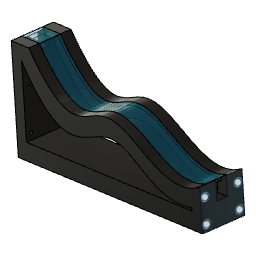
Light Fight Enclosurev2 (Autodesk Fusion 360 archive; units mm, degrees)
design "curvy ramp v4"
Autodesk Fusion 360 part; units mm, degrees
sketch "Sketch1" plane through (0, 0, 0) normal (0, 0, 1) x (1, 0, 0)
  spline S0 degree 5 poles (40.5611, 35.8703) (42.6613, 34.7671) (46.8791, 32.8536) (53.2584, 30.8623) (61.8698, 29.9771) (72.8022, 31.7845) (83.8683, 36.2451) (94.9958, 42.7502) (106.047, 50.0933) (116.8416, 56.5913) (127.2385, 60.6523) (137.2101, 61.2633) (146.9114, 58.4588) (156.7874, 54.0175) (167.5021, 51.0733) (179.7981, 53.3109) (191.4637, 62.1139) (201.4823, 73.9015) (208.7561, 84.2233) (212.5417, 90) knots 0 0 0 0 0 0 0.066667 0.133333 0.2 0.266667 0.333333 0.4 0.466667 0.533333 0.6 0.666667 0.733333 0.8 0.866667 0.933333 1 1 1 1 1 1
  line L0 (179.6056, 39.7401) -> (245.4778, 140.2599)
  line L1 (220.9765, 77.3947) -> (220.9765, 14.5028)
  line L2 (220.9765, 14.5028) -> (50.4348, 14.5028)
  line L3 (40.5611, -0.1297) -> (230.5611, -0.1297)
  line L4 (230.5611, -0.1297) -> (230.5611, 90)
  line L5 (230.5611, 90) -> (220.5417, 90)
  line L6 (212.5417, 90) -> (220.5417, 90)
  line L7 (40.5611, -0.1297) -> (40.5611, 35.8703)
  line L8 (50.4348, 25) -> (50.4348, 29.3921)
  line L9 (45.8578, 33.4692) -> (45.8578, 30.6235)
  spline S1 degree 5 poles (50.4348, 19.7514) (52.5108, 19.1803) (56.647, 18.3263) (62.8042, 17.9102) (70.9306, 19.0395) (81.008, 22.9144) (91.0643, 28.6518) (101.1393, 35.3853) (111.2165, 41.8888) (121.2381, 46.7548) (131.17, 48.8392) (141.0534, 47.6422) (151.0639, 43.7411) (161.5707, 39.2349) (173.0583, 37.1534) (186.051, 40.8954) (198.0379, 51.1114) (208.0885, 63.9297) (215.2808, 74.9049) (219, 81) knots 0 0 0 0 0 0 0.066667 0.133333 0.2 0.266667 0.333333 0.4 0.466667 0.533333 0.6 0.666667 0.733333 0.8 0.866667 0.933333 1 1 1 1 1 1
  line L10 (32.1895, 24.771) -> (68.6802, 14.7318)
  line L11 (195.2279, 42.0418) -> (242.7721, 119.9582)
  spline S2 degree 5 poles (50.4348, 16.9226) (52.4566, 16.5812) (56.4561, 16.0582) (62.3233, 15.7536) (69.8813, 16.311) (78.8871, 18.5852) (87.4629, 22.3093) (95.6403, 27.1967) (103.4817, 32.7308) (111.0884, 38.1119) (118.5816, 42.4668) (126.0845, 45.0565) (133.7053, 45.4599) (141.516, 43.8367) (149.5484, 40.9252) (157.8085, 37.7615) (166.2855, 35.4806) (174.9622, 35.0844) (183.8241, 37.2318) (192.8599, 42.3179) (202.0608, 50.5417) (209.5491, 59.6846) (215.2356, 67.9819) (219.0577, 74.1509) (220.9765, 77.3947) knots 0 0 0 0 0 0 0.05 0.1 0.15 0.2 0.25 0.3 0.35 0.4 0.45 0.5 0.55 0.6 0.65 0.7 0.75 0.8 0.85 0.9 0.95 1 1 1 1 1 1
  line L12 (50.4348, 14.5028) -> (50.4348, 16.9226)
  line L13 (50.4348, 19.7514) -> (50.4348, 25)
  line L14 (215.1059, 87.8623) -> (225.0015, 87.8623)
  line L15 (219, 87.8623) -> (219, 81)
  spline S3 degree 5 poles (45.8578, 30.6235) (46.8345, 30.3152) (48.8626, 29.7261) (51.9972, 28.9749) (56.3314, 28.2647) (62.0148, 27.9438) (68.063, 28.3589) (74.4833, 29.7325) (81.3346, 32.2418) (88.6448, 35.9334) (96.3871, 40.6346) (104.4508, 45.8412) (112.6696, 50.8468) (120.8567, 54.9054) (128.8386, 57.3848) (136.4873, 57.9163) (143.7577, 56.569) (150.7125, 53.9616) (157.4785, 51.0206) (164.2106, 48.7743) (171.0561, 48.1534) (178.1115, 49.7453) (185.4085, 53.7203) (192.9378, 59.985) (200.3861, 67.977) (206.3983, 75.5527) (210.881, 81.718) (213.7908, 85.9219) (215.1059, 87.8623) knots 0.042086 0.042086 0.042086 0.042086 0.042086 0.042086 0.08 0.12 0.16 0.2 0.24 0.28 0.32 0.36 0.4 0.44 0.48 0.52 0.56 0.6 0.64 0.68 0.72 0.76 0.8 0.84 0.88 0.92 0.96 0.992837 0.992837 0.992837 0.992837 0.992837 0.992837
  line L16 (27.6195, 36.3811) -> (64.096, 24.866)
  line L17 (199.2828, 64.5154) -> (230.9291, 111.2092)
  line L18 (225.0015, 90) -> (225.0015, 87.8623)
  line L19 (219, 81) -> (230.5611, 81)
  line L20 (50.4348, 29.3921) -> (40.5611, 29.3921)
  line L21 (50.4348, 19.7514) -> (40.5611, 19.7514)
  line L22 (225.0015, 87.8623) -> (230.5611, 87.8623)
  point P0 (90, 40)
  point P1 (140, 60)
  point P2 (169.2008, 69.6255)
  point P3 (141, 47)
  point P4 (96, 32)
  point P5 (59.8517, 28.1591)
  point P6 (89.7554, 36.7453)
  point P7 (135.1987, 57.4887)
  point P8 (168.0748, 48.6766)
  point P9 (95, 27)
  point P10 (130, 45)
  point P11 (166, 36)
  dimension "d1" = 36
  dimension "d2" = 8
  dimension "d3" = 190
  constraint vertical L7
  constraint horizontal L6
  constraint perpendicular L3 L7
  constraint perpendicular L3 L4
  constraint perpendicular L4 L5
  constraint perpendicular L1 L5
  constraint perpendicular L1 L2
  constraint perpendicular L2 L12
  constraint midpoint S0.end L0
  constraint parallel L8 L12
  constraint coincident S0 L9.start
  constraint vertical L9
  constraint coincident L8.end S3
  constraint coincident S1.start L12
  constraint midpoint S1.start L10
  constraint midpoint S1.end L11
  constraint collinear L12 L13
  constraint perpendicular L4 L14
  constraint coincident L14 L15.start
  constraint midpoint L9.end L16
  constraint midpoint L14.start L17
  constraint coincident L5 L18.start
  constraint perpendicular L14 L18
  constraint coincident L4 L19.end
  constraint perpendicular L4 L19
  constraint coincident L7 L20.end
  constraint perpendicular L7 L20
  constraint coincident L7 L21.end
  constraint coincident L4 L22.end
  constraint perpendicular L4 L22
  measures "d1" distance of L3.start S0.start
  measures "d2" distance of S0.end L5.end
  measures "d3" distance of L3.start L3.end
extrude "Extrude5" add sketch "Sketch1" along normal blind 40 contours S0 L7 L9 L16 | S0 L0 L9 S3 | L7 L16 L20 | L0 L6 S3 L17 | S3 L16 L20 | L7 L8 L10 L13 L16 L20 | L0 S1 L14 L15 S3 | L0 L8 S1 L13 S3 | L5 L6 L11 L14 L17 | L8 L16 L20 | L7 L10 L21 | S1 L10 L11 S2 | L1 L2 L3 L4 L7 L10 L11 S2 L12 L19 L21 | L11 L14 L15 | L4 L11 L14 L19 L22 | L5 L11 L14 L18 | L4 L5 L18 L22 makes body 1
extrude "Extrude6" cut sketch "Sketch1" along normal blind 30 contours S0 L0 L9 S3 | L0 L6 S3 L17 | L0 S1 L14 L15 S3 | L0 L8 S1 L13 S3 | L5 L6 L11 L14 L17 | L5 L11 L14 L18 bodies 1
extrude "Extrude7" cut sketch "Sketch1" along normal blind 25 contours S0 L7 L9 L16 | L7 L16 L20 | S3 L16 L20 | L7 L8 L10 L13 L16 L20 | L8 L16 L20 | L7 L10 L21 | L11 L14 L15 | L4 L11 L14 L19 L22 | L4 L5 L18 L22 bodies 1
extrude "Extrude8" add sketch "Sketch1" along normal blind 15 contours S0 L7 L9 L16 | L7 L16 L20 | S3 L16 L20 | L7 L8 L10 L13 L16 L20 | L8 L16 L20 | L7 L10 L21 | L11 L14 L15 | L4 L11 L14 L19 L22 | L4 L5 L18 L22 bodies 1
extrude "Extrude9" add sketch "Sketch1" along normal blind 10 contours S0 L0 L9 S3 | L0 L6 S3 L17 | L0 S1 L14 L15 S3 | L0 L8 S1 L13 S3 | L5 L6 L11 L14 L17 | L5 L11 L14 L18 bodies 1
extrude "Extrude11" cut sketch "Sketch1" along normal blind 30 contours L4 L5 L18 L22 bodies 1
extrude "Extrude12" add sketch "Sketch1" along normal blind 10 contours L4 L5 L18 L22 bodies 1
extrude "Extrude13" add sketch "Sketch1" along normal blind 20 separate body contours S0 L0 L9 S3 | L0 L6 S3 L17 | L5 L6 L11 L14 L17 | L5 L11 L14 L18 | L4 L5 L18 L22 makes body 2
move_body "Move6" bodies 2 to x (1, 0, 0) y (0, 1, 0) z (0, 0, 1) at (0, 0, 10)
sketch "Sketch2" plane through (40.5611, 0, 0) normal (-1, 0, 0) x (0, -1, 0)
  line L0 (-35.8703, 25) -> (-19.7514, 25)
  line L1 (-19.7514, 25) -> (-19.7514, 15)
  line L2 (-19.7514, 15) -> (-35.8703, 15)
  line L3 (-35.8703, 15) -> (-35.8703, 0)
  line L4 (-35.8703, 0) -> (0.1297, 0)
  line L5 (0.1297, 0) -> (0.1297, 40)
  line L6 (0.1297, 40) -> (-35.8703, 40)
  line L7 (-35.8703, 40) -> (-35.8703, 25)
  circle A0 centre (-27, 4) radius 2.95
  circle A1 centre (-27.0541, 35.3502) radius 2.95
  circle A2 centre (-6, 4) radius 2.95
  circle A3 centre (-6.0541, 35.3502) radius 2.95
  dimension "d34" = 5.9
  dimension "d35" = 5.9
  dimension "d36" = 5.9
  dimension "d37" = 5.9
  measures "d34" diameter of A0
  measures "d35" diameter of A1
  measures "d36" diameter of A2
  measures "d37" diameter of A3
extrude "Extrude14" cut sketch "Sketch2" against normal blind 2.4 contours A0 | A1 | A2 | A3 bodies 1
sketch "Sketch3" plane through (230.5611, 0, 0) normal (1, 0, 0) x (0, 1, 0)
  line L0 (87.8623, 10) -> (87.8623, 15)
  line L1 (87.8623, 15) -> (81, 15)
  line L2 (81, 15) -> (81, 25)
  line L3 (81, 25) -> (87.8623, 25)
  line L4 (87.8623, 25) -> (87.8623, 30)
  line L5 (87.8623, 30) -> (90, 30)
  line L6 (90, 30) -> (90, 40)
  line L7 (90, 40) -> (-0.1297, 40)
  line L8 (-0.1297, 40) -> (-0.1297, 0)
  line L9 (-0.1297, 0) -> (90, 0)
  line L10 (90, 0) -> (90, 10)
  line L11 (90, 10) -> (87.8623, 10)
  circle A0 centre (55, 35) radius 2.95
  circle A1 centre (55, 35) radius 2.95
  circle A2 centre (55, 35) radius 1.5
  circle A3 centre (55, 35) radius 1.5
  circle A4 centre (55, 5) radius 2.95
  circle A5 centre (55, 5) radius 2.95
  circle A6 centre (55, 5) radius 1.5
  circle A7 centre (55, 5) radius 1.5
  circle A8 centre (20, 35) radius 2.95
  circle A9 centre (20, 35) radius 2.95
  circle A10 centre (20, 35) radius 1.5
  circle A11 centre (20, 35) radius 1.5
  circle A12 centre (20, 5) radius 1.5
  circle A13 centre (20, 5) radius 1.5
  circle A14 centre (20, 5) radius 2.95
  circle A15 centre (20, 5) radius 2.95
  point P0 (55, 35)
  point P1 (55, 35)
  point P2 (55, 5)
  point P3 (55, 5)
  point P4 (20, 35)
  point P5 (20, 35)
  point P6 (20, 5)
  point P7 (20, 5)
  dimension "d40" = 5.9
  dimension "d41" = 5.9
  dimension "d45" = 3
  dimension "d46" = 3
  dimension "d47" = 5.9
  dimension "d48" = 5.9
  dimension "d49" = 3
  dimension "d50" = 3
  dimension "d51" = 5.9
  dimension "d52" = 5.9
  dimension "d53" = 3
  dimension "d54" = 3
  dimension "d55" = 5.9
  dimension "d56" = 5.9
  dimension "d57" = 3
  dimension "d58" = 3
  constraint concentric A0 A2
  constraint concentric A4 A6
  constraint concentric A8 A10
  constraint concentric A12 A14
  measures "d40" diameter of A0
  measures "d41" diameter of A1
  measures "d45" diameter of A2
  measures "d46" diameter of A3
  measures "d47" diameter of A4
  measures "d48" diameter of A5
  measures "d49" diameter of A6
  measures "d50" diameter of A7
  measures "d51" diameter of A8
  measures "d52" diameter of A9
  measures "d53" diameter of A10
  measures "d54" diameter of A11
  measures "d55" diameter of A14
  measures "d56" diameter of A15
  measures "d57" diameter of A12
  measures "d58" diameter of A13
extrude "Extrude15" cut sketch "Sketch3" against normal blind 2.4 contours A0 A1 | A2 A3 | A4 A5 | A6 A7 | A8 A9 | A10 A11 | A12 A13 | A14 A15 bodies 1
extrude "Extrude16" cut sketch "Sketch3" against normal blind 10 contours A2 A3 | A6 A7 | A10 A11 | A12 A13 bodies 1
equation "neopixelwidth = 20 mm"
equation "sidethickness = 10 mm"
equation "d30 = neopixelwidth"
equation "magneddiam = 5.9 mm"
equation "magnetDepth = 2.4 mm"
equation "d34 = magneddiam"
equation "d35 = magneddiam"
equation "d36 = magneddiam"
equation "d37 = magneddiam"
equation "d38 = -magnetDepth"
equation "d40 = magneddiam"
equation "d41 = magneddiam"
equation "d47 = magneddiam"
equation "d48 = magneddiam"
equation "d51 = magneddiam"
equation "d52 = magneddiam"
equation "d55 = magneddiam"
equation "d56 = magneddiam"
equation "d59 = -magnetDepth"
named bodies: "blackPLA", "clearPLA"
